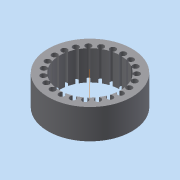
# Autodesk Inventor part: Сердечник корпуса
Saved by Autodesk Inventor 2016 SP1 (Build 200210100, 210)
## iProperties
Created: 2016-05-17
Part Number: Сердечник корпуса
Material: Сталь, ковкая
Document SubType Name: Modeling
Designer: a.kaluzhenin
Density: 7.85 g/cm^3
Appearance: Сталь
Mass: 3160.33 g
Surface Area: 952.806 cm^2
Volume: 402.589 cm^3
Author: a.kaluzhenin
Autodesk Inventor part; units mm, degrees
ref_plane "YZ Plane" through (0, 0, 0) normal (1, 0, 0) x (0, 1, 0)
ref_plane "XZ Plane" through (0, 0, 0) normal (0, 1, 0) x (-1, 0, 0)
ref_plane "XY Plane" through (0, 0, 0) normal (0, 0, 1) x (1, 0, 0)
sketch "Эскиз1" plane through (0, 0, 0) normal (0, 0, 1) x (1, 0, 0)
  circle A0 centre (0, 0) radius 81 construction
  circle A1 centre (0, 0) radius 55 construction
  circle A2 centre (0, 0) radius 79
  line L0 (0, 57.0002) -> (0, 68) construction
  arc A3 (2.5, 57.6012) -> (-2.5295, 57.6164) centre (0, 62.5001) ccw
  line L1 (2.5, 56.9451) -> (2.5, 57.6012)
  line L2 (-2.5, 56.9451) -> (-2.5295, 57.6164)
  line L3 (-15.3785, 54.8865) -> (-18.3462, 65.4784) construction
  arc A4 (-13.1333, 56.1397) -> (-17.9804, 54.7973) centre (-16.8623, 60.1824) ccw
  line L4 (-12.9563, 55.508) -> (-13.1333, 56.1397)
  line L5 (-17.7709, 54.159) -> (-17.9804, 54.7973)
  line L6 (-29.6164, 48.7021) -> (-35.3317, 58.1005) construction
  arc A5 (-27.7926, 50.5146) -> (-32.0978, 47.9143) centre (-32.474, 53.4013) ccw
  line L7 (-27.4517, 49.954) -> (-27.7926, 50.5146)
  line L8 (-31.7238, 47.3561) -> (-32.0978, 47.9143)
  line L9 (-41.6578, 38.9056) -> (-49.6968, 46.4136) construction
  arc A6 (-40.3907, 41.143) -> (-43.8346, 37.4776) centre (-45.6773, 42.6596) ccw
  line L10 (-39.9112, 40.6952) -> (-40.3907, 41.143)
  line L11 (-43.3239, 37.041) -> (-43.8346, 37.4776)
  line L12 (-50.6096, 26.2238) -> (-60.3762, 31.2844) construction
  arc A7 (-49.9931, 28.72) -> (-52.3204, 24.2614) centre (-55.4929, 28.7541) ccw
  line L13 (-49.4106, 28.4182) -> (-49.9931, 28.72)
  line L14 (-51.7109, 23.9788) -> (-52.3204, 24.2614)
  line L15 (-55.808, 11.597) -> (-66.5777, 13.835) construction
  arc A8 (-55.8878, 14.167) -> (-56.9259, 9.2458) centre (-61.1928, 12.716) ccw
  line L16 (-55.2454, 14.0335) -> (-55.8878, 14.167)
  line L17 (-56.2627, 9.1381) -> (-56.9259, 9.2458)
  line L18 (-56.8673, -3.8898) -> (-67.8415, -4.6405) construction
  arc A9 (-57.6375, -1.4367) -> (-57.3094, -6.4554) centre (-62.3544, -4.2652) ccw
  line L19 (-56.983, -1.3919) -> (-57.6375, -1.4367)
  line L20 (-56.6418, -6.3802) -> (-57.3094, -6.4554)
  line L21 (-53.709, -19.0882) -> (-64.0737, -22.7718) construction
  arc A10 (-55.1126, -16.9338) -> (-53.4426, -21.678) centre (-58.8914, -20.93) ccw
  line L22 (-54.4944, -16.7141) -> (-55.1126, -16.9338)
  line L23 (-52.82, -21.4254) -> (-53.4426, -21.678)
  line L24 (-46.5674, -32.8709) -> (-55.554, -39.2143) construction
  arc A11 (-48.5002, -31.1751) -> (-45.6121, -35.2927) centre (-51.0607, -36.0426) ccw
  line L25 (-47.9642, -30.7967) -> (-48.5002, -31.1751)
  line L26 (-45.0808, -34.8816) -> (-45.6121, -35.2927)
  line L27 (-35.9721, -44.2157) -> (-42.914, -52.7484) construction
  arc A12 (-38.2907, -43.1042) -> (-34.3989, -46.29) centre (-39.4431, -48.482) ccw
  line L28 (-37.8767, -42.5953) -> (-38.2907, -43.1042)
  line L29 (-33.9981, -45.7507) -> (-34.3989, -46.29)
  line L30 (-22.7089, -52.2812) -> (-27.0913, -62.3704) construction
  arc A13 (-25.2414, -51.8365) -> (-20.6344, -53.8541) centre (-24.9001, -57.3258) ccw
  line L31 (-24.98, -51.2347) -> (-25.2414, -51.8365)
  line L32 (-20.394, -53.2267) -> (-20.6344, -53.8541)
  line L33 (-7.7615, -56.4693) -> (-9.2593, -67.3666) construction
  arc A14 (-10.3201, -56.7243) -> (-5.3395, -57.4241) centre (-8.5104, -61.918) ccw
  line L34 (-10.2307, -56.0743) -> (-10.3201, -56.7243)
  line L35 (-5.2773, -56.7552) -> (-5.3395, -57.4241)
  line L36 (7.7615, -56.4693) -> (9.2593, -67.3666) construction
  arc A15 (5.3666, -57.4051) -> (10.3513, -56.7353) centre (8.5104, -61.918) ccw
  line L37 (5.2773, -56.7552) -> (5.3666, -57.4051)
  line L38 (10.2307, -56.0743) -> (10.3513, -56.7353)
  line L39 (22.7089, -52.2812) -> (27.0913, -62.3704) construction
  arc A16 (20.6554, -53.8285) -> (25.2745, -51.8386) centre (24.9001, -57.3258) ccw
  line L40 (20.394, -53.2267) -> (20.6554, -53.8285)
  line L41 (24.98, -51.2347) -> (25.2745, -51.8386)
  line L42 (35.9721, -44.2157) -> (42.914, -52.7484) construction
  arc A17 (34.4121, -46.2596) -> (38.3231, -43.0973) centre (39.4431, -48.482) ccw
  line L43 (33.9981, -45.7507) -> (34.4121, -46.2596)
  line L44 (37.8767, -42.5953) -> (38.3231, -43.0973)
  line L45 (46.5674, -32.8709) -> (55.554, -39.2143) construction
  arc A18 (45.6168, -35.2599) -> (48.5295, -31.1597) centre (51.0607, -36.0426) ccw
  line L46 (45.0808, -34.8816) -> (45.6168, -35.2599)
  line L47 (47.9642, -30.7967) -> (48.5295, -31.1597)
  line L48 (53.709, -19.0882) -> (64.0737, -22.7718) construction
  arc A19 (53.4382, -21.6451) -> (55.1367, -16.9111) centre (58.8914, -20.93) ccw
  line L49 (52.82, -21.4254) -> (53.4382, -21.6451)
  line L50 (54.4944, -16.7141) -> (55.1367, -16.9111)
  line L51 (56.8673, -3.8898) -> (67.8415, -4.6405) construction
  arc A20 (57.2963, -6.425) -> (57.6547, -1.4083) centre (62.3544, -4.2652) ccw
  line L52 (56.6418, -6.3802) -> (57.2963, -6.425)
  line L53 (56.983, -1.3919) -> (57.6547, -1.4083)
  line L54 (55.808, 11.597) -> (66.5777, 13.835) construction
  arc A21 (56.9051, 9.2716) -> (55.8966, 14.199) centre (61.1928, 12.716) ccw
  line L55 (56.2627, 9.1381) -> (56.9051, 9.2716)
  line L56 (55.2454, 14.0335) -> (55.8966, 14.199)
  line L57 (50.6096, 26.2238) -> (60.3762, 31.2844) construction
  arc A22 (52.2934, 24.2806) -> (49.993, 28.7531) centre (55.4929, 28.7541) ccw
  line L58 (51.7109, 23.9788) -> (52.2934, 24.2806)
  line L59 (49.4106, 28.4182) -> (49.993, 28.7531)
  line L60 (41.6578, 38.9056) -> (49.6968, 46.4136) construction
  arc A23 (43.8034, 37.4888) -> (40.3816, 41.1749) centre (45.6773, 42.6596) ccw
  line L61 (43.3239, 37.041) -> (43.8034, 37.4888)
  line L62 (39.9112, 40.6952) -> (40.3816, 41.1749)
  line L63 (29.6164, 48.7021) -> (35.3317, 58.1005) construction
  arc A24 (32.0647, 47.9166) -> (27.7753, 50.5428) centre (32.474, 53.4013) ccw
  line L64 (31.7238, 47.3561) -> (32.0647, 47.9166)
  line L65 (27.4517, 49.954) -> (27.7753, 50.5428)
  line L66 (15.3785, 54.8865) -> (18.3462, 65.4784) construction
  arc A25 (17.9479, 54.7907) -> (13.109, 56.1622) centre (16.8623, 60.1824) ccw
  line L67 (17.7709, 54.159) -> (17.9479, 54.7907)
  line L68 (12.9563, 55.508) -> (13.109, 56.1622)
  arc A26 (12.9563, 55.508) -> (2.5, 56.9451) centre (0, 0) ccw
  arc A27 (27.4517, 49.954) -> (17.7709, 54.159) centre (0, 0) ccw
  arc A28 (39.9112, 40.6952) -> (31.7238, 47.3561) centre (0, 0) ccw
  arc A29 (49.4106, 28.4182) -> (43.3239, 37.041) centre (0, 0) ccw
  arc A30 (55.2454, 14.0335) -> (51.7109, 23.9788) centre (0, 0) ccw
  arc A31 (56.983, -1.3919) -> (56.2627, 9.1381) centre (0, 0) ccw
  arc A32 (54.4944, -16.7141) -> (56.6418, -6.3802) centre (0, 0) ccw
  arc A33 (47.9642, -30.7967) -> (52.82, -21.4254) centre (0, 0) ccw
  arc A34 (37.8767, -42.5953) -> (45.0808, -34.8816) centre (0, 0) ccw
  arc A35 (24.98, -51.2347) -> (33.9981, -45.7507) centre (0, 0) ccw
  arc A36 (10.2307, -56.0743) -> (20.394, -53.2267) centre (0, 0) ccw
  arc A37 (-5.2773, -56.7552) -> (5.2773, -56.7552) centre (0, 0) ccw
  arc A38 (-20.394, -53.2267) -> (-10.2307, -56.0743) centre (0, 0) ccw
  arc A39 (-33.9981, -45.7507) -> (-24.98, -51.2347) centre (0, 0) ccw
  arc A40 (-45.0808, -34.8816) -> (-37.8767, -42.5953) centre (0, 0) ccw
  arc A41 (-52.82, -21.4254) -> (-47.9642, -30.7967) centre (0, 0) ccw
  arc A42 (-56.6418, -6.3802) -> (-54.4944, -16.7141) centre (0, 0) ccw
  arc A43 (-56.2627, 9.1381) -> (-56.983, -1.3919) centre (0, 0) ccw
  arc A44 (-51.7109, 23.9788) -> (-55.2454, 14.0335) centre (0, 0) ccw
  arc A45 (-43.3239, 37.041) -> (-49.4106, 28.4182) centre (0, 0) ccw
  arc A46 (-31.7238, 47.3561) -> (-39.9112, 40.6952) centre (0, 0) ccw
  arc A47 (-2.5, 56.9451) -> (-12.9563, 55.508) centre (0, 0) ccw
  arc A48 (-17.7709, 54.159) -> (-27.4517, 49.954) centre (0, 0) ccw
  point P0 (0, 0)
  point P1 (2.5, 56.9451)
  point P2 (-12.9563, 55.508)
  point P3 (-27.4517, 49.954)
  point P4 (-39.9112, 40.6952)
  point P5 (-49.4106, 28.4182)
  point P6 (-55.2454, 14.0335)
  point P7 (-56.983, -1.3919)
  point P8 (-54.4944, -16.7141)
  point P9 (-47.9642, -30.7967)
  point P10 (-37.8767, -42.5953)
  point P11 (-24.98, -51.2347)
  point P12 (-10.2307, -56.0743)
  point P13 (5.2773, -56.7552)
  point P14 (20.394, -53.2267)
  point P15 (33.9981, -45.7507)
  point P16 (45.0808, -34.8816)
  point P17 (52.82, -21.4254)
  point P18 (56.6418, -6.3802)
  point P19 (56.2627, 9.1381)
  point P20 (51.7109, 23.9788)
  point P21 (43.3239, 37.041)
  point P22 (31.7238, 47.3561)
  point P23 (17.7709, 54.159)
  dimension "d0" = 2
  dimension "d7" = 5.4999
  dimension "d8" = 2.5
  dimension "d11" = 360
  constraints: 138 end point, 92 point on circle, 47 centre point, 24 coincident, 23 line through centre, 23 point on line, 1 midpoint, 1 parallel, 1 symmetric about line, 1 vertical, 1 vertical alignment, 575 other
  measures "d0" radial gap between concentric circles of A0 A2
  measures "d7" radius of A3
  measures "d8" distance between parallel lines of L1 L0
extrude "Выдавливание1" add sketch "Эскиз1" along normal mid plane 56
